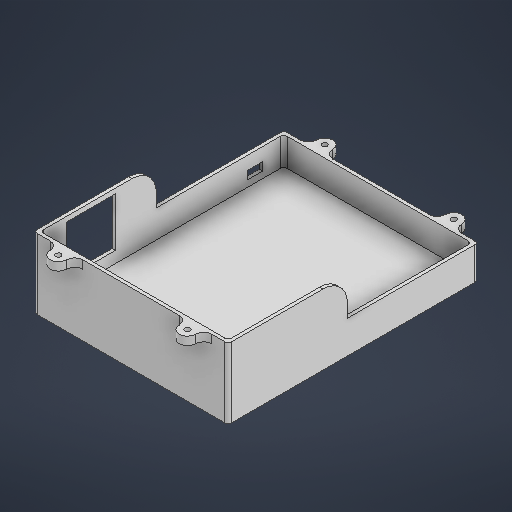
# Autodesk Inventor part: base
Saved by Autodesk Inventor 2026.1 (Build 301233020, 233B)
## iProperties
Created: 2026-06-29
Part Number: base
Material: Generic
Document SubType Name: Modeling
Designer: Asus
Density: 1 g/cm^3
Appearance: Default
Author: Asus
Autodesk Inventor part; units mm, degrees
ref_plane "YZ Plane" through (0, 0, 0) normal (1, 0, 0) x (0, 1, 0)
ref_plane "XZ Plane" through (0, 0, 0) normal (0, 1, 0) x (-1, 0, 0)
ref_plane "XY Plane" through (0, 0, 0) normal (0, 0, 1) x (1, 0, 0)
sketch "Sketch2" plane through (0, 0, 0) normal (0, 1, 0) x (-1, 0, 0)
  line L0 (0, 0) -> (119, 0)
  line L1 (119, 0) -> (119, -153)
  line L2 (119, -153) -> (0, -153)
  line L3 (0, -153) -> (0, 0)
  dimension "d0" = 119
  dimension "d1" = 153
  constraints: 8 end point, 2 parallel, 1 horizontal, 1 perpendicular
  measures "d0" distance of L1.end L2.end
  measures "d1" distance of L0.end L1.end
extrude "Extrusion1" add sketch "Sketch2" along normal blind 3
sketch "Sketch7" plane through (0, 3, 0) normal (0, 1, 0) x (1, 0, 0)
  line L0 (-117, 2) -> (-2, 2)
  line L1 (-2, 2) -> (-2, 151)
  line L2 (-2, 151) -> (-117, 151)
  line L3 (-117, 151) -> (-117, 2)
  line L4 (-119, 153) -> (-119, 0) projected
  line L5 (-119, 0) -> (0, 0) projected
  line L6 (0, 153) -> (-119, 153) projected
  line L7 (-119, 0) -> (0, 0)
  line L8 (0, 0) -> (0, 153)
  line L9 (0, 153) -> (-119, 153)
  line L10 (-119, 153) -> (-119, 0)
  dimension "d27" = 115
  dimension "d28" = 149
  dimension "d29" = 2
  dimension "d30" = 2
  constraints: 16 end point, 4 parallel, 2 horizontal, 2 perpendicular
  measures "d27" distance of L2.end L1.end
  measures "d28" distance of L1.end L0.end
  measures "d29" distance between parallel lines of L3 L4
  measures "d30" distance between parallel lines of L5 L0
extrude "Extrusion5" add sketch "Sketch7" along normal blind 17
sketch "Sketch8" plane through (0, 20, 0) normal (0, 1, 0) x (1, 0, 0)
  line L0 (-119, 0) -> (0, 0) projected
  line L1 (-119, 0) -> (0, 0)
  line L2 (0, 0) -> (0, 73)
  line L3 (-119, 73) -> (-119, 0)
  line L4 (-117, 2) -> (-117, 151) projected
  line L5 (-2, 151) -> (-2, 2) projected
  line L6 (-117, 2) -> (-2, 2)
  line L7 (-2, 2) -> (-2, 73)
  line L8 (-2, 73) -> (-117, 73)
  line L9 (-117, 73) -> (-117, 2)
  line L10 (0, 73) -> (-2, 73)
  line L11 (-117, 73) -> (-119, 73)
  dimension "d33" = 119
  dimension "d34" = 73
  constraints: 18 end point, 5 parallel, 2 horizontal, 2 perpendicular, 2 point on line
  measures "d33" distance of L3.start L2.end
  measures "d34" distance of L2.end L1.end
extrude "Extrusion6" add sketch "Sketch8" along normal blind 23 contours L3 L11 L4 L6 L5 L10 L2 L0
sketch "Sketch9" plane through (-119, 0, -153) normal (-1, 0, 0) x (0, 0, 1)
  line L0 (15, 12) -> (24, 12)
  line L1 (24, 12) -> (24, 7)
  line L2 (24, 7) -> (15, 7)
  line L3 (15, 7) -> (15, 12)
  line L4 (2, 3) -> (151, 3) projected
  line L5 (0, 0) -> (0, 20) projected
  line L6 (2, 3) -> (2, 20) projected
  line L7 (105, 40) -> (135, 40)
  line L8 (135, 40) -> (135, 10)
  line L9 (135, 10) -> (105, 10)
  line L10 (105, 10) -> (105, 40)
  line L11 (0, 0) -> (153, 0) projected
  line L12 (80, 20) -> (80, 43) projected
  dimension "d37" = 9
  dimension "d38" = 5
  dimension "d39" = 4
  dimension "d40" = 15
  dimension "d41" = 13
  dimension "d42" = 30
  dimension "d43" = 30
  dimension "d44" = 10
  dimension "d45" = 25
  constraints: 16 end point, 4 parallel, 2 horizontal, 2 perpendicular
  measures "d37" distance of L1.end L2.end
  measures "d38" distance of L0.end L1.end
  measures "d39" distance between parallel lines of L2 L4
  measures "d40" distance between parallel lines of L3 L5
  measures "d41" distance between parallel lines of L6 L3
  measures "d42" distance of L8.end L9.end
  measures "d43" distance of L7.end L8.end
  measures "d44" distance between parallel lines of L11 L9
  measures "d45" distance between parallel lines of L10 L12
extrude "Extrusion7" cut sketch "Sketch9" against normal blind 23
fillet "Fillet1" radius 2 8 edges at (-119, 10, -153) (-117, 11.5, -151) (0, 21.5, 0) (0, 10, -153) (-119, 21.5, 0) (-2, 23, -2) (-2, 11.5, -151) (-117, 23, -2)
fillet "Fillet2" radius 15 2 edges at (-118, 43, -73) (-1, 43, -73)
sketch "Sketch10" plane through (-117, 0, 0) normal (0, 0, 1) x (1, 0, 0)
  line L0 (113, 43) -> (2, 43) projected
  line L1 (13, 43) -> (23, 43)
  line L2 (23, 43) -> (23, 38)
  line L3 (23, 38) -> (13, 38)
  line L4 (13, 38) -> (13, 43)
  line L5 (92, 43) -> (102, 43)
  line L6 (102, 43) -> (102, 38)
  line L7 (102, 38) -> (92, 38)
  line L8 (92, 38) -> (92, 43)
  line L9 (117, 0) -> (117, 43) projected
  line L10 (-2, 43) -> (-2, 0) projected
  point P0 (23, 43)
  dimension "d50" = 10
  dimension "d51" = 5
  dimension "d52" = 10
  dimension "d53" = 5
  dimension "d54" = 119
  dimension "d55" = 15
  dimension "d56" = 15
  constraints: 16 end point, 4 parallel, 2 horizontal, 2 perpendicular, 2 point on line
  measures "d50" distance of L2.end L3.end
  measures "d51" distance of L1.end L2.end
  measures "d52" distance of L6.end L7.end
  measures "d53" distance of L5.end L6.end
  measures "d54" distance between parallel lines of L9 L10
  measures "d55" distance between parallel lines of L4 L10
  measures "d56" distance between parallel lines of L9 L6
extrude "Extrusion8" add sketch "Sketch10" along normal blind 10
sketch "Sketch11" plane through (-2, 0, -153) normal (0, 0, -1) x (-1, 0, 0)
  line L0 (113, 20) -> (2, 20) projected
  line L1 (13, 20) -> (23, 20)
  line L2 (23, 20) -> (23, 15)
  line L3 (23, 15) -> (13, 15)
  line L4 (13, 15) -> (13, 20)
  line L5 (92, 20) -> (102, 20)
  line L6 (102, 20) -> (102, 15)
  line L7 (102, 15) -> (92, 15)
  line L8 (92, 15) -> (92, 20)
  line L9 (-2, 20) -> (-2, 0) projected
  line L10 (117, 0) -> (117, 20) projected
  dimension "d59" = 10
  dimension "d60" = 5
  dimension "d61" = 10
  dimension "d62" = 5
  dimension "d63" = 15
  dimension "d64" = 15
  constraints: 16 end point, 4 parallel, 2 horizontal, 2 perpendicular, 2 point on line
  measures "d59" distance of L2.end L3.end
  measures "d60" distance of L1.end L2.end
  measures "d61" distance of L6.end L7.end
  measures "d62" distance of L5.end L6.end
  measures "d63" distance between parallel lines of L4 L9
  measures "d64" distance between parallel lines of L10 L6
extrude "Extrusion9" add sketch "Sketch11" along normal blind 10
sketch "Sketch12" plane through (0, 43, 0) normal (0, 1, 0) x (1, 0, 0)
  circle A0 centre (-99, -5) radius 1.65
  line L0 (-94, -10) -> (-104, -10) projected
  circle A1 centre (-20, -5) radius 1.65
  line L1 (-15, -10) -> (-25, -10) projected
  line L2 (-104, 0) -> (-104, -10) projected
  line L3 (-15, 0) -> (-15, -10) projected
  point P0 (0, 0)
  dimension "d67" = 3.3
  dimension "d68" = 5
  dimension "d69" = 3.3
  dimension "d70" = 5
  dimension "d71" = 5
  dimension "d72" = 5
  constraints: 2 centre point
  measures "d67" diameter of A0
  measures "d68" distance from line of A0.centre L0
  measures "d69" diameter of A1
  measures "d70" distance from line of A1.centre L1
  measures "d71" distance from line of A0.centre L2
  measures "d72" distance from line of A1.centre L3
extrude "Extrusion10" cut sketch "Sketch12" against normal blind 10
sketch "Sketch13" plane through (0, 20, 0) normal (0, 1, 0) x (1, 0, 0)
  circle A0 centre (-99, 158) radius 1.65
  line L0 (-104, 153) -> (-104, 163) projected
  line L1 (-104, 163) -> (-94, 163) projected
  circle A1 centre (-20, 158) radius 1.65
  line L2 (-25, 153) -> (-25, 163) projected
  line L3 (-25, 163) -> (-15, 163) projected
  point P0 (0, 0)
  point P1 (-25, 158)
  dimension "d75" = 3.3
  dimension "d76" = 5
  dimension "d77" = 5
  dimension "d78" = 3.3
  dimension "d79" = 5
  dimension "d80" = 5
  constraints: 2 centre point, 1 midpoint
  measures "d75" diameter of A0
  measures "d76" distance from line of A0.centre L0
  measures "d77" distance from line of A0.centre L1
  measures "d78" diameter of A1
  measures "d79" distance of point (-25, 158) A1.centre
  measures "d80" distance from line of A1.centre L3
extrude "Extrusion11" cut sketch "Sketch13" against normal blind 10
fillet "Fillet3" radius 5 16 edges at (-15, 17.5, -163) (-25, 17.5, -163) (-15, 17.5, -153) (-94, 17.5, -163) (-94, 17.5, -153) (-25, 17.5, -153) (-104, 17.5, -163) (-104, 17.5, -153) (-104, 40.5, 0) (-104, 40.5, 10) (-94, 40.5, 10) (-94, 40.5, 0) (-25, 40.5, 10) (-15, 40.5, 10) (-15, 40.5, 0) (-25, 40.5, 0)
body "Solid1"
